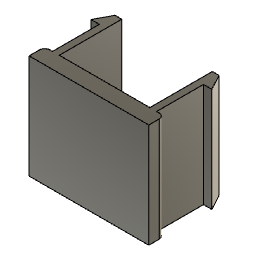
Kabelführung_Boschprofil (Autodesk Fusion 360 design; units mm, degrees)
Autodesk Fusion 360 part; units mm, degrees
sketch "Skizze1" plane through (0, 0, 0) normal (0, 0, 1) x (1, 0, 0)
  line L0 (0, 0) -> (-5.75, 0)
  line L1 (-5.75, 0) -> (-5.75, 1.5)
  line L2 (-5.75, 1.5) -> (-5, 1.5)
  line L3 (-5, 1.5) -> (-5, 6)
  line L4 (-5, 6) -> (-5.8, 6)
  line L5 (-5.8, 6) -> (-5, 7.5)
  line L6 (-5, 7.5) -> (-4.35, 7.5)
  line L7 (-4.35, 7.5) -> (-4.35, 1.5)
  line L8 (-4.35, 1.5) -> (0, 1.5)
  line L9 (0, 1.5) -> (0, 0)
  line L10 (0, 2.5) -> (0, 20)
  line L11 (0, 0) -> (5.75, 0)
  line L12 (5.75, 0) -> (5.75, 1.5)
  line L13 (5.75, 1.5) -> (5, 1.5)
  line L14 (5, 6) -> (5.8, 6)
  line L15 (5.8, 6) -> (5, 7.5)
  line L16 (5, 7.5) -> (4.35, 7.5)
  line L17 (4.35, 1.5) -> (0, 1.5)
  line L18 (0, 1.5) -> (0, 0)
  line L19 (5, 1.5) -> (5, 6)
  line L20 (4.35, 7.5) -> (4.35, 1.5)
  dimension "d1" = 1.5
  dimension "d2" = 1.5
  dimension "d3" = 1.5
  dimension "d4" = 7.5
  dimension "d5" = 5.75
  dimension "d6" = 4.35
  dimension "d7" = 5.8
  dimension "d8" = 5
  dimension "d10" = 0.65
  constraint coincident L0.start L9.end
  constraint horizontal L0
  constraint perpendicular L0 L1
  constraint perpendicular L1 L2
  constraint perpendicular L2 L3
  constraint perpendicular L3 L4
  constraint parallel L2 L6
  constraint perpendicular L6 L7
  constraint perpendicular L7 L8
  constraint perpendicular L0 L9
  constraint symmetric L0.start L10 L9.end
  constraint symmetric L0.end L10 L11.end
  constraint symmetric L1.end L10 L12.end
  constraint symmetric L2.end L10 L13.end
  constraint symmetric L3.end L10 L14.start
  constraint symmetric L4.end L10 L14.end
  constraint symmetric L5.end L10 L15.end
  constraint symmetric L6.end L10 L16.end
  constraint symmetric L7.end L10 L17.start
  constraint symmetric L8.end L10 L9.start
  measures "d1" distance of L8.end L0.start
  measures "d2" distance of L0.end L1.end
  measures "d3" distance of L4 L6
  measures "d4" distance of L0 L6
  measures "d5" distance of L0.start L0.end
  measures "d6" distance of L7.end L8.end
  measures "d7" horizontal distance of L0.start L4.end
  measures "d8" distance of L0.start L3
  measures "d10" distance of L5.end L6.end
extrude "Extrusion1" add sketch "Skizze1" along normal blind 10
fillet "Abrundung1" radius 0.5 2 edges at (5.75, 1.5, 5) (-5.75, 1.5, 5)
equation "d5 = ( 11.5 / 2 ) * 1 mm"
equation "d6 = ( 8.7 / 2 ) * 1 mm"
equation "d7 = ( 11.6 / 2 ) * 1 mm"
equation "d10 = d8 - d6"
